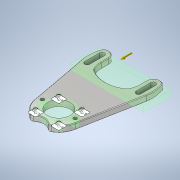
# Autodesk Inventor part: Motor Holder v3
Saved by Autodesk Inventor 2020.1 (Build 241239000, 239)
## iProperties
Created: 2019-03-01
Part Number: Motor Holder v3
Material: Aluminum 6061-AHC
Document SubType Name: Modeling
Designer: Petar
Density: 2.7 g/cm^3
Appearance: Aluminum - Dark
Mass: 29.5264 g
Surface Area: 65.3151 cm^2
Volume: 10.9357 cm^3
Author: Petar
Autodesk Inventor part; units mm, degrees
ref_plane "YZ Plane" through (0, 0, 0) normal (1, 0, 0) x (0, 1, 0)
ref_plane "XZ Plane" through (0, 0, 0) normal (0, 1, 0) x (-1, 0, 0)
ref_plane "XY Plane" through (0, 0, 0) normal (0, 0, 1) x (1, 0, 0)
sketch "Sketch1" plane through (0, 0, 0) normal (0, 1, 0) x (-1, 0, 0)
  line L0 (0, 0) -> (0, 51.5) construction
  circle A0 centre (0, 51.5) radius 9.5
  line L1 (16, -6.25) -> (16, 0)
  line L2 (21.5, 19.9197) -> (21.5, -14.0803) construction
  line L3 (-21.5, 18) -> (-21.5, -16) construction
  circle A1 centre (21.5, 3.5) radius 1.75 construction
  circle A2 centre (21.5, -3.5) radius 1.75 construction
  circle A3 centre (-21.5, 3.5) radius 1.75 construction
  circle A4 centre (-21.5, -3.5) radius 1.75 construction
  line L4 (-16, -6.25) -> (-16, 0)
  line L5 (21.5, 6.25) -> (21.5, -6.25) construction
  line L6 (19.45, 6.25) -> (19.45, -6.25)
  line L7 (23.55, -6.25) -> (23.55, 6.25)
  arc A5 (23.55, 6.25) -> (19.45, 6.25) centre (21.5, 6.25) ccw
  arc A6 (19.45, -6.25) -> (23.55, -6.25) centre (21.5, -6.25) ccw
  line L8 (-19.45, 6.25) -> (-19.45, -6.25)
  line L9 (-23.55, -6.25) -> (-23.55, 6.25)
  arc A7 (-19.45, 6.25) -> (-23.55, 6.25) centre (-21.5, 6.25) ccw
  arc A8 (-23.55, -6.25) -> (-19.45, -6.25) centre (-21.5, -6.25) ccw
  arc A9 (14.5447, 41.7686) -> (17.1997, 54.7282) centre (0, 51.5) ccw construction
  arc A10 (16, -6.25) -> (24.816, -10.638) centre (21.5, -6.25) ccw
  arc A11 (-24.816, -10.638) -> (-16, -6.25) centre (-21.5, -6.25) ccw
  line L10 (17.1997, 54.7282) -> (26.5367, 4.9806)
  line L11 (-17.1997, 54.7282) -> (-26.5367, 4.9806)
  circle A12 centre (0, 51.5) radius 13.75 construction
  circle A13 centre (9.7227, 61.2227) radius 1.5
  circle A14 centre (9.7227, 41.7773) radius 1.5
  line L12 (0, 51.5) -> (9.7227, 61.2227) construction
  line L13 (9.7227, 41.7773) -> (0, 51.5) construction
  circle A15 centre (-9.7227, 61.2227) radius 1.5
  circle A16 centre (-9.7227, 41.7773) radius 1.5
  circle A17 centre (13.75, 51.5) radius 1.5
  line L14 (13.75, 51.5) -> (0, 51.5) construction
  circle A18 centre (-13.75, 51.5) radius 1.5
  circle A19 centre (0, 22.9421) radius 1.5 construction
  line L15 (14.5447, 41.7686) -> (18.7351, 19.4421) construction
  arc A20 (17.1997, 54.7282) -> (-17.1997, 54.7282) centre (0, 51.5) ccw
  arc A21 (-17.1997, 54.7282) -> (-14.5447, 41.7686) centre (0, 51.5) ccw construction
  line L16 (-14.5447, 41.7686) -> (-18.7351, 19.4421) construction
  line L17 (7.5, 67.3114) -> (0, 61) construction
  line L18 (0, 61) -> (-7.5, 67.3114) construction
  spline S0 degree 2 poles (7.5, 67.3114) (0, 61) (-7.5, 67.3114) knots 1 1 1 2 2 2
  line L19 (7.5, 67.3114) -> (-7.5, 67.3114) construction
  line L20 (18.7351, 19.4421) -> (-18.7351, 19.4421) construction
  line L21 (18.7351, 19.4421) -> (11.8062, 33.8844) construction
  line L22 (14.5447, 41.7686) -> (12.1087, 38.1277) construction
  arc A22 (12.1087, 38.1277) -> (11.8062, 33.8844) centre (15.676, 35.7409) ccw construction
  line L23 (-18.7351, 19.4421) -> (-11.8062, 33.8844) construction
  line L24 (-14.5447, 41.7686) -> (-12.1087, 38.1277) construction
  arc A23 (-11.8062, 33.8844) -> (-12.1087, 38.1277) centre (-15.676, 35.7409) ccw construction
  line L25 (14.2986, 19.4421) -> (8.1631, 32.2306) construction
  line L26 (14.2986, 19.4421) -> (7.4946, 25.939) construction
  line L27 (8.1631, 32.2306) -> (6.9952, 30.485) construction
  arc A24 (6.9952, 30.485) -> (7.4946, 25.939) centre (9.9486, 28.509) ccw construction
  line L28 (-14.2986, 19.4421) -> (-8.1631, 32.2306) construction
  line L29 (-14.2986, 19.4421) -> (-7.4946, 25.939) construction
  line L30 (-8.1631, 32.2306) -> (-6.9952, 30.485) construction
  arc A25 (-7.4946, 25.939) -> (-6.9952, 30.485) centre (-9.9486, 28.509) ccw construction
  arc A26 (24.816, -10.638) -> (27, 0) centre (0, 0) ccw
  arc A27 (-24.816, -10.638) -> (24.816, -10.638) centre (0, 0) ccw construction
  arc A28 (-10.2709, 24.9702) -> (-26.5367, 4.9806) centre (0, 0) ccw construction
  line L31 (21.5, -11.75) -> (-21.5, -11.75) construction
  line L32 (-21.2132, 69) -> (25, 69) construction
  line L33 (0, 61) -> (0, 61) construction
  arc A29 (13.761, 8.163) -> (-13.761, 8.163) centre (0, -11.5) ccw
  line L34 (13.761, 8.163) -> (-13.761, 8.163) construction
  arc A30 (16, 0) -> (13.761, 8.163) centre (0, 0) ccw
  arc A31 (-13.761, 8.163) -> (-16, 0) centre (0, 0) ccw
  arc A32 (27, 0) -> (26.5367, 4.9806) centre (0, 0) ccw
  arc A33 (-27, 0) -> (-24.816, -10.638) centre (0, 0) ccw
  arc A34 (-26.5367, 4.9806) -> (-27, 0) centre (0, 0) ccw
  arc A35 (26.5367, 4.9806) -> (-12.0292, 24.1722) centre (0, 0) ccw construction
  line L35 (16, 0) -> (-16, 0) construction
  point P0 (21.5, 0)
  point P1 (0, 12.5)
  dimension "d1" = 19
  dimension "d0" = 51.5
  dimension "d3" = 3.5
  dimension "d4" = 3.5
  dimension "d5" = 7
  dimension "d9" = 3.5
  dimension "d11" = 32
  dimension "d15" = 4.1
  dimension "d24" = 3
  dimension "d25" = 3
  dimension "d27" = 45
  dimension "d29" = 3
  dimension "d30" = 3
  dimension "d50" = 15
  dimension "d53" = 27
  dimension "d75" = 80.75
  dimension "d76" = 8
  dimension "d78" = 0
  dimension "d81" = 6.25
  dimension "d82" = 12.5
  dimension "d85" = 5
  dimension "d86" = 4
  dimension "d98" = 15
  dimension "d99" = 24
  dimension "d101" = 43
  dimension "d104" = 2
  dimension "d105" = 27.5
  constraints: 70 end point, 58 point on circle, 35 centre point, 26 symmetric about line, 19 tangent, 13 point on line, 7 coincident, 5 horizontal, 5 vertical, 3 parallel, 2 perpendicular, 1 collinear, 1 midpoint, 1 vertical alignment, 16 other
  measures "d0" distance of L0.start L0.end
  measures "d3" diameter of A1
  measures "d4" diameter of A2
  measures "d5" distance of A2.centre A1.centre
  measures "d9" vertical distance of L0.start A1.centre
  measures "d11" distance between parallel lines of L4 L1
  measures "d15" distance between parallel lines of L6 L7
  measures "d24" diameter of A13
  measures "d25" diameter of A14
  measures "d27" angle of L0 L13
  measures "d29" diameter of A17
  measures "d30" diameter of A19
  measures "d50" distance of L17.start L18.end
  measures "d53" radius of A26
  measures "d75" distance between parallel lines of L31 L32
  measures "d78" distance of L33.start L33.end
  measures "d81" vertical distance of L5.start point (0, 12.5)
  measures "d82" distance of L5.end L5.start
  measures "d85" distance between parallel lines of L10 L15
  measures "d86" distance between parallel lines of L21 L25
  measures "d98" angle of L15 L21
  measures "d99" radius of A29
  measures "d101" distance of A4.centre A2.centre
  measures "d104" distance edge to line of A19 L20
  measures "d105" diameter of A12
extrude "Extrusion3" add sketch "Sketch1" along normal blind 5 contours L1 A30 A29 A31 L4 A11 A33 A34 L11 A20 S0 L10 A32 A26 A10
thread "Thread1" size "M3x0.5" class "6H" standard "ANSI Metric M Profile" full length
thread "Thread2" size "M3x0.5" class "6H" standard "ANSI Metric M Profile" full length
thread "Thread4" size "M3x0.5" class "6H" standard "ANSI Metric M Profile" full length
thread "Thread5" size "M3x0.5" class "6H" standard "ANSI Metric M Profile" full length
thread "Thread6" size "M3x0.5" class "6H" standard "ANSI Metric M Profile" full length
thread "Thread7" size "M3x0.5" class "6H" standard "ANSI Metric M Profile" full length
sketch "Sketch3" plane through (0, 5, 0) normal (0, 1, 0) x (1, 0, 0)
  line L0 (0, 0) -> (0, -51.5) construction
  circle A0 centre (0, -51.5) radius 9.5 construction
  arc A1 (-24.816, 10.638) -> (-26.5367, -4.9806) centre (0, 0) ccw construction
  line L1 (-7.003, -18.2122) -> (-6.6985, -18.2122)
  line L2 (-7.003, -14.735) -> (-7.003, -18.2122)
  line L3 (-6.6985, -18.2122) -> (-6.6985, -14.735)
  spline S0 degree 3 poles (-5.654, -15.6487) (-5.6375, -15.9355) (-5.5157, -16.1411) (-5.2606, -16.3086) knots 0 0 0 0 1 1 1 1
  spline S1 degree 3 poles (-5.0436, -16.0662) (-5.3012, -15.8898) (-5.3888, -15.6005) (-5.2759, -15.2997) knots 0 0 0 0 1 1 1 1
  spline S2 degree 3 poles (-5.2759, -15.2997) (-5.2175, -15.1423) (-5.0411, -15.0078) (-4.8266, -14.9558) knots 0 0 0 0 1 1 1 1
  spline S3 degree 3 poles (-4.8583, -14.6842) (-5.3723, -14.768) (-5.6832, -15.1436) (-5.654, -15.6487) knots 0 0 0 0 1 1 1 1
  spline S4 degree 3 poles (-4.7441, -14.6652) (-4.7543, -14.6677) (-4.8063, -14.6766) (-4.8583, -14.6842) knots 0 0 0 0 1 1 1 1
  line L4 (-6.6985, -14.735) -> (-7.003, -14.735)
  line L5 (-9.7696, -16.702) -> (-9.4485, -16.702)
  spline S5 degree 3 poles (-9.4485, -16.702) (-8.9497, -16.702) (-8.6731, -16.669) (-8.4294, -16.5814) knots 0 0 0 0 1 1 1 1
  line L6 (-10.0741, -14.7324) -> (-10.0741, -18.2122)
  line L7 (-9.7696, -18.2122) -> (-9.7696, -16.702)
  line L8 (-10.0741, -18.2122) -> (-9.7696, -18.2122)
  spline S6 degree 3 poles (-7.8457, -15.9418) (-7.8165, -15.7946) (-7.8266, -15.5193) (-7.866, -15.3822) knots 0 0 0 0 1 1 1 1
  spline S7 degree 3 poles (-8.4294, -16.5814) (-8.1084, -16.4672) (-7.9066, -16.2464) (-7.8457, -15.9418) knots 0 0 0 0 1 1 1 1
  spline S8 degree 3 poles (-7.866, -15.3822) (-7.965, -15.0383) (-8.1997, -14.8543) (-8.6439, -14.7718) knots 0 0 0 0 1 1 1 1
  spline S9 degree 3 poles (-8.1617, -15.6487) (-8.1426, -15.9609) (-8.2568, -16.1868) (-8.4916, -16.301) knots 0 0 0 0 1 1 1 1
  spline S10 degree 3 poles (-8.6236, -15.0624) (-8.3178, -15.1462) (-8.1832, -15.3187) (-8.1617, -15.6487) knots 0 0 0 0 1 1 1 1
  spline S11 degree 3 poles (-8.4916, -16.301) (-8.6782, -16.3936) (-8.8127, -16.4101) (-9.366, -16.4101) knots 0 0 0 0 1 1 1 1
  line L9 (-9.366, -16.4101) -> (-9.7696, -16.4101)
  line L10 (-9.7696, -16.4101) -> (-9.7696, -15.0243)
  spline S12 degree 3 poles (-4.5284, -16.301) (-4.6305, -16.2646) (-4.7394, -16.2225) (-4.9041, -16.1474) (-4.9836, -16.1078) (-5.0436, -16.0662) knots -1.508252 -1.508252 -1.508252 -1.508252 -0.608749 -0.608749 0 0 0 0
  spline S13 degree 3 poles (-5.2606, -16.3086) (-5.1261, -16.3974) (-4.9599, -16.4698) (-4.5982, -16.5954) knots 0 0 0 0 1 1 1 1
  line L11 (-5.4078, -17.3111) -> (-5.7353, -17.3111)
  line L12 (-5.7353, -17.3111) -> (-5.7264, -17.3708)
  line L13 (-5.3875, -17.4101) -> (-5.4078, -17.3111)
  spline S14 degree 3 poles (-4.8266, -14.9558) (-4.7061, -14.9253) (-4.4205, -14.9266) (-4.2809, -14.9558) knots 0 0 0 0 1 1 1 1
  spline S15 degree 3 poles (-4.2289, -14.6893) (-4.3215, -14.6715) (-4.6972, -14.6538) (-4.7441, -14.6652) knots 0 0 0 0 1 1 1 1
  line L14 (-3.8012, -15.405) -> (-3.786, -15.4837)
  spline S16 degree 3 poles (-4.2809, -14.9558) (-4.0106, -15.0142) (-3.8469, -15.169) (-3.8012, -15.405) knots 0 0 0 0 1 1 1 1
  line L15 (-3.786, -15.4837) -> (-3.4738, -15.4837)
  line L16 (-3.4738, -15.4837) -> (-3.4827, -15.4355)
  spline S17 degree 3 poles (-3.4827, -15.4355) (-3.5233, -15.1982) (-3.5817, -15.07) (-3.7086, -14.9431) knots 0 0 0 0 1 1 1 1
  spline S18 degree 3 poles (-3.7086, -14.9431) (-3.8456, -14.8073) (-3.9903, -14.7363) (-4.2289, -14.6893) knots 0 0 0 0 1 1 1 1
  spline S19 degree 3 poles (-1.4344, -14.6779) (-1.8812, -14.7502) (-2.2187, -15.0066) (-2.4281, -15.4304) knots 0 0 0 0 1 1 1 1
  spline S20 degree 3 poles (-2.3202, -16.4736) (-2.3202, -15.683) (-2.0144, -15.1373) (-1.4877, -14.9863) knots 0 0 0 0 1 1 1 1
  spline S21 degree 3 poles (-1.4877, -14.9863) (-1.4027, -14.9621) (-1.357, -14.9571) (-1.1908, -14.9571) knots 0 0 0 0 1 1 1 1
  spline S22 degree 3 poles (-1.1908, -14.9571) (-1.0195, -14.9571) (-0.9814, -14.9609) (-0.8989, -14.9863) knots 0 0 0 0 1 1 1 1
  spline S23 degree 3 poles (-0.8532, -14.6956) (-0.9916, -14.6614) (-1.2834, -14.6525) (-1.4344, -14.6779) knots 0 0 0 0 1 1 1 1
  line L17 (-0.3862, -15.5116) -> (-0.3786, -15.5472)
  spline S24 degree 3 poles (-0.8989, -14.9863) (-0.6121, -15.0776) (-0.4446, -15.2489) (-0.3862, -15.5116) knots 0 0 0 0 1 1 1 1
  spline S25 degree 3 poles (-0.1882, -15.1233) (-0.3266, -14.9127) (-0.5461, -14.7705) (-0.8532, -14.6956) knots 0 0 0 0 1 1 1 1
  spline S26 degree 3 poles (-0.0537, -15.4812) (-0.069, -15.3708) (-0.1261, -15.2185) (-0.1882, -15.1233) knots 0 0 0 0 1 1 1 1
  line L18 (-0.3786, -15.5472) -> (-0.0448, -15.5472)
  line L19 (-0.0448, -15.5472) -> (-0.0537, -15.4812)
  spline S27 degree 3 poles (-2.4281, -15.4304) (-2.6451, -15.8695) (-2.7086, -16.4774) (-2.5944, -17.0332) knots 0 0 0 0 1 1 1 1
  spline S28 degree 3 poles (-5.2365, -17.7401) (-5.3, -17.6614) (-5.3634, -17.5231) (-5.3875, -17.4101) knots 0 0 0 0 1 1 1 1
  spline S29 degree 3 poles (-5.7264, -17.3708) (-5.6997, -17.5535) (-5.6071, -17.7794) (-5.5056, -17.9051) knots 0 0 0 0 1 1 1 1
  spline S30 degree 3 poles (-4.7746, -17.9914) (-4.8679, -17.9737) (-4.9599, -17.9443) (-5.1175, -17.8586) (-5.1837, -17.8061) (-5.2365, -17.7401) knots -1.494677 -1.494677 -1.494677 -1.494677 -0.705114 -0.705114 0 0 0 0
  spline S31 degree 3 poles (-5.5056, -17.9051) (-5.305, -18.1538) (-4.9561, -18.2883) (-4.5094, -18.2883) knots 0 0 0 0 1 1 1 1
  spline S32 degree 3 poles (-9.2454, -15.0294) (-8.7581, -15.0345) (-8.7162, -15.037) (-8.6236, -15.0624) knots 0 0 0 0 1 1 1 1
  spline S33 degree 3 poles (-8.6439, -14.7718) (-8.7721, -14.7477) (-8.847, -14.7439) (-9.4294, -14.7388) knots 0 0 0 0 1 1 1 1
  line L20 (-9.4294, -14.7388) -> (-10.0741, -14.7324)
  line L21 (-9.7696, -15.0243) -> (-9.2454, -15.0294)
  spline S34 degree 3 poles (-0.7314, -17.8936) (-0.8862, -17.9711) (-0.9751, -17.9901) (-1.1908, -17.9901) knots 0 0 0 0 1 1 1 1
  spline S35 degree 3 poles (-0.3862, -17.4342) (-0.4306, -17.6373) (-0.5588, -17.8061) (-0.7314, -17.8936) knots 0 0 0 0 1 1 1 1
  spline S36 degree 3 poles (-1.1083, -18.2832) (-0.6997, -18.2629) (-0.3672, -18.0967) (-0.1882, -17.8238) knots 0 0 0 0 1 1 1 1
  line L22 (-0.3786, -17.4) -> (-0.3862, -17.4342)
  line L23 (-0.0461, -17.4) -> (-0.3786, -17.4)
  line L24 (-0.055, -17.466) -> (-0.0461, -17.4)
  spline S37 degree 3 poles (-0.1882, -17.8238) (-0.1261, -17.7287) (-0.0702, -17.5776) (-0.055, -17.466) knots 0 0 0 0 1 1 1 1
  line L25 (1.1569, -14.735) -> (0.8524, -14.735)
  line L26 (1.1569, -16.2578) -> (1.1569, -14.735)
  line L27 (0.8524, -14.735) -> (0.8524, -18.2122)
  line L28 (0.8524, -18.2122) -> (1.1569, -18.2122)
  line L29 (1.1569, -18.2122) -> (1.1569, -16.5497)
  line L30 (1.1569, -16.5497) -> (3.0224, -16.5497)
  line L31 (3.0224, -16.2578) -> (1.1569, -16.2578)
  line L32 (5.1786, -16.4025) -> (5.9413, -15.5751)
  line L33 (4.8055, -16.3543) -> (4.8017, -15.5446)
  spline S38 degree 3 poles (6.7027, -14.7413) (6.7027, -14.7375) (6.6177, -14.735) (6.5149, -14.735) knots 0 0 0 0 1 1 1 1
  spline S39 degree 3 poles (5.9413, -15.5751) (6.36, -15.1195) (6.7027, -14.7439) (6.7027, -14.7413) knots 0 0 0 0 1 1 1 1
  line L34 (6.5149, -14.735) -> (6.3258, -14.735)
  line L35 (6.3258, -14.735) -> (4.8055, -16.3543)
  line L36 (4.8017, -15.5446) -> (4.7991, -14.735)
  line L37 (3.327, -14.735) -> (3.0224, -14.735)
  line L38 (4.7991, -14.735) -> (4.4945, -14.735)
  line L39 (3.0224, -14.735) -> (3.0224, -16.2578)
  line L40 (5.2344, -16.4596) -> (5.1786, -16.4025)
  spline S40 degree 3 poles (6.0174, -17.3048) (5.6176, -16.8721) (5.2649, -16.4913) (5.2344, -16.4596) knots 0 0 0 0 1 1 1 1
  line L41 (4.8017, -17.3568) -> (4.8055, -16.5002)
  line L42 (4.4945, -14.735) -> (4.4945, -18.2122)
  line L43 (3.327, -18.2122) -> (3.327, -14.735)
  line L44 (4.8055, -16.5002) -> (6.4298, -18.2109)
  line L45 (3.0224, -16.5497) -> (3.0224, -18.2122)
  line L46 (3.0224, -18.2122) -> (3.327, -18.2122)
  line L47 (4.4945, -18.2122) -> (4.7991, -18.2122)
  line L48 (4.7991, -18.2122) -> (4.8017, -17.3568)
  line L49 (6.4298, -18.2109) -> (6.6456, -18.2122)
  spline S41 degree 3 poles (6.8029, -18.1513) (6.7699, -18.1183) (6.4171, -17.7375) (6.0174, -17.3048) knots 0 0 0 0 1 1 1 1
  line L50 (6.86, -18.2122) -> (6.8029, -18.1513)
  line L51 (6.6456, -18.2122) -> (6.86, -18.2122)
  spline S42 degree 3 poles (8.3892, -14.7629) (8.3829, -14.7794) (8.0783, -15.5599) (7.7116, -16.499) knots 0 0 0 0 1 1 1 1
  spline S43 degree 3 poles (8.1976, -16.0053) (8.5695, -15.0345) (8.5745, -15.0243) (8.591, -15.0662) knots 0 0 0 0 1 1 1 1
  spline S44 degree 3 poles (8.5796, -14.735) (8.4083, -14.735) (8.4019, -14.7363) (8.3892, -14.7629) knots 0 0 0 0 1 1 1 1
  line L52 (8.756, -14.735) -> (8.5796, -14.735)
  line L53 (8.8524, -14.9786) -> (8.756, -14.735)
  spline S45 degree 3 poles (8.591, -15.0662) (8.6012, -15.089) (8.8182, -15.6652) (9.0758, -16.3467) knots 0 0 0 0 1 1 1 1
  spline S46 degree 3 poles (9.5314, -16.7147) (9.2103, -15.8949) (8.9057, -15.1132) (8.8524, -14.9786) knots 0 0 0 0 1 1 1 1
  spline S47 degree 3 poles (7.7573, -17.1652) (7.7915, -17.0675) (7.9908, -16.5459) (8.1976, -16.0053) knots 0 0 0 0 1 1 1 1
  line L54 (7.0479, -18.2058) -> (7.2001, -18.2096)
  spline S48 degree 3 poles (7.2001, -18.2096) (7.2839, -18.2109) (7.3562, -18.2109) (7.3588, -18.2071) knots 0 0 0 0 1 1 1 1
  line L55 (7.7116, -16.499) -> (7.0479, -18.2058)
  spline S49 degree 3 poles (7.3588, -18.2071) (7.3677, -18.1982) (7.6824, -17.3746) (7.7573, -17.1652) knots 0 0 0 0 1 1 1 1
  spline S50 degree 3 poles (-4.1934, -17.9774) (-4.3101, -18.0104) (-4.6324, -18.018) (-4.7746, -17.9914) knots 0 0 0 0 1 1 1 1
  ellipse E0 centre (-21.8716, 1.388) end of major axis (-3.6125, -17.9928) minor radius 4.9544 (-4.5094, -18.2883) -> (-3.8558, -18.1589) ccw
  spline S51 degree 3 poles (-3.8558, -18.1589) (-3.7695, -18.117) (-3.7276, -18.0865) (-3.6451, -18.004) knots 0 0 0 0 1 1 1 1
  spline S52 degree 3 poles (-3.7327, -17.3924) (-3.753, -17.7084) (-3.9015, -17.8962) (-4.1934, -17.9774) knots 0 0 0 0 1 1 1 1
  spline S53 degree 3 poles (-3.6451, -18.004) (-3.4789, -17.8378) (-3.4154, -17.6779) (-3.4027, -17.3924) knots 0 0 0 0 1 1 1 1
  spline S54 degree 3 poles (-4.5982, -16.5954) (-4.2644, -16.7109) (-4.1464, -16.7604) (-4.0284, -16.834) knots 0 0 0 0 1 1 1 1
  spline S55 degree 3 poles (-3.951, -16.5281) (-4.0626, -16.4723) (-4.1743, -16.4292) (-4.5284, -16.301) knots 0 0 0 0 1 1 1 1
  spline S56 degree 3 poles (-1.1908, -17.9901) (-1.357, -17.9901) (-1.4027, -17.985) (-1.4877, -17.9609) knots 0 0 0 0 1 1 1 1
  spline S57 degree 3 poles (-1.4877, -17.9609) (-2.0144, -17.8099) (-2.3202, -17.2629) (-2.3202, -16.4736) knots 0 0 0 0 1 1 1 1
  spline S58 degree 3 poles (-2.5944, -17.0332) (-2.423, -17.8632) (-1.8761, -18.3226) (-1.1083, -18.2832) knots 0 0 0 0 1 1 1 1
  spline S59 degree 3 poles (-3.4167, -17.1297) (-3.4751, -16.8683) (-3.6413, -16.6817) (-3.951, -16.5281) knots 0 0 0 0 1 1 1 1
  spline S60 degree 3 poles (-4.0284, -16.834) (-3.8076, -16.971) (-3.7162, -17.1449) (-3.7327, -17.3924) knots 0 0 0 0 1 1 1 1
  spline S61 degree 3 poles (-3.4027, -17.3924) (-3.3977, -17.2617) (-3.4002, -17.2058) (-3.4167, -17.1297) knots 0 0 0 0 1 1 1 1
  line L56 (8.204, -17.9203) -> (8.1532, -18.0637)
  line L57 (8.1532, -18.0637) -> (8.1037, -18.2058)
  line L58 (8.1037, -18.2058) -> (8.6012, -18.2096)
  line L59 (8.9362, -17.9178) -> (8.204, -17.9203)
  spline S62 degree 3 poles (9.0758, -16.3467) (9.3334, -17.0269) (9.572, -17.6576) (9.6063, -17.749) knots 0 0 0 0 1 1 1 1
  line L60 (9.6697, -17.9139) -> (8.9362, -17.9178)
  spline S63 degree 3 poles (8.6012, -18.2096) (8.8753, -18.2109) (9.3271, -18.2109) (9.6063, -18.2096) knots 0 0 0 0 1 1 1 1
  line L61 (9.6063, -17.749) -> (9.6697, -17.9139)
  line L62 (9.6063, -18.2096) -> (10.1139, -18.2058)
  line L63 (10.1139, -18.2058) -> (9.5314, -16.7147)
  point P0 (0, -22.9421)
  constraints: 128 end point, 2 coincident, 2 horizontal alignment, 1 vertical, 194 other
emboss "Emboss1" [suppressed]
sketch "Sketch4" plane through (0, 0, 0) normal (0, -1, 0) x (1, 0, 0)
  circle A0 centre (0, 51.5) radius 9.5 construction
  arc A1 (24.816, -10.638) -> (26.5367, 4.9806) centre (0, 0) ccw construction
  line L0 (0, 0) -> (0, 51.5) construction
  spline S0 degree 3 poles (8.013, 15.7172) (7.9838, 15.57) (7.994, 15.2946) (8.0333, 15.1575) knots 0 0 0 0 1 1 1 1
  spline S1 degree 3 poles (8.5968, 16.3568) (8.2757, 16.2425) (8.0739, 16.0217) (8.013, 15.7172) knots 0 0 0 0 1 1 1 1
  spline S2 degree 3 poles (8.329, 15.424) (8.31, 15.7362) (8.4242, 15.9621) (8.6589, 16.0763) knots 0 0 0 0 1 1 1 1
  spline S3 degree 3 poles (8.7909, 14.8377) (8.4851, 14.9215) (8.3506, 15.0941) (8.329, 15.424) knots 0 0 0 0 1 1 1 1
  spline S4 degree 3 poles (8.0333, 15.1575) (8.1323, 14.8136) (8.3671, 14.6296) (8.8112, 14.5471) knots 0 0 0 0 1 1 1 1
  spline S5 degree 3 poles (9.6158, 16.4773) (9.1171, 16.4773) (8.8404, 16.4443) (8.5968, 16.3568) knots 0 0 0 0 1 1 1 1
  line L1 (9.9369, 16.4773) -> (9.6158, 16.4773)
  line L2 (9.9369, 17.9875) -> (9.9369, 16.4773)
  line L3 (10.2414, 17.9875) -> (9.9369, 17.9875)
  line L4 (10.2414, 14.5078) -> (10.2414, 17.9875)
  spline S6 degree 3 poles (8.6589, 16.0763) (8.8455, 16.1689) (8.98, 16.1854) (9.5333, 16.1854) knots 0 0 0 0 1 1 1 1
  line L5 (9.5333, 16.1854) -> (9.9369, 16.1854)
  spline S7 degree 3 poles (9.4128, 14.8047) (8.9254, 14.8098) (8.8836, 14.8123) (8.7909, 14.8377) knots 0 0 0 0 1 1 1 1
  line L6 (9.9369, 16.1854) -> (9.9369, 14.7996)
  spline S8 degree 3 poles (8.8112, 14.5471) (8.9394, 14.523) (9.0143, 14.5192) (9.5968, 14.5141) knots 0 0 0 0 1 1 1 1
  line L7 (9.9369, 14.7996) -> (9.4128, 14.8047)
  line L8 (9.5968, 14.5141) -> (10.2414, 14.5078)
  spline S9 degree 3 poles (4.9114, 14.4405) (4.9216, 14.443) (4.9736, 14.4519) (5.0257, 14.4595) knots 0 0 0 0 1 1 1 1
  spline S10 degree 3 poles (4.9939, 14.7311) (4.8734, 14.7007) (4.5878, 14.7019) (4.4482, 14.7311) knots 0 0 0 0 1 1 1 1
  spline S11 degree 3 poles (3.8759, 14.7184) (4.013, 14.5826) (4.1576, 14.5116) (4.3962, 14.4646) knots 0 0 0 0 1 1 1 1
  spline S12 degree 3 poles (4.3962, 14.4646) (4.4889, 14.4468) (4.8645, 14.4291) (4.9114, 14.4405) knots 0 0 0 0 1 1 1 1
  spline S13 degree 3 poles (4.4482, 14.7311) (4.1779, 14.7895) (4.0142, 14.9443) (3.9685, 15.1804) knots 0 0 0 0 1 1 1 1
  line L9 (3.9685, 15.1804) -> (3.9533, 15.259)
  spline S14 degree 3 poles (4.1183, 16.3035) (4.23, 16.2476) (4.3416, 16.2045) (4.6957, 16.0763) knots 0 0 0 0 1 1 1 1
  spline S15 degree 3 poles (4.7655, 16.3707) (4.4317, 16.4862) (4.3137, 16.5357) (4.1957, 16.6093) knots 0 0 0 0 1 1 1 1
  line L10 (3.9533, 15.259) -> (3.6411, 15.259)
  line L11 (3.6411, 15.259) -> (3.65, 15.2108)
  spline S16 degree 3 poles (3.584, 16.905) (3.6424, 16.6436) (3.8086, 16.457) (4.1183, 16.3035) knots 0 0 0 0 1 1 1 1
  spline S17 degree 3 poles (4.1957, 16.6093) (3.9749, 16.7464) (3.8835, 16.9202) (3.9, 17.1677) knots 0 0 0 0 1 1 1 1
  spline S18 degree 3 poles (3.5701, 17.1677) (3.565, 17.037) (3.5675, 16.9811) (3.584, 16.905) knots 0 0 0 0 1 1 1 1
  spline S19 degree 3 poles (1.6018, 14.4532) (2.0485, 14.5255) (2.386, 14.7819) (2.5954, 15.2057) knots 0 0 0 0 1 1 1 1
  spline S20 degree 3 poles (2.5954, 15.2057) (2.8124, 15.6448) (2.8759, 16.2527) (2.7617, 16.8085) knots 0 0 0 0 1 1 1 1
  spline S21 degree 3 poles (2.4876, 16.2489) (2.4876, 15.4583) (2.1817, 14.9126) (1.6551, 14.7616) knots 0 0 0 0 1 1 1 1
  spline S22 degree 3 poles (3.8125, 17.7794) (3.6462, 17.6131) (3.5828, 17.4532) (3.5701, 17.1677) knots 0 0 0 0 1 1 1 1
  spline S23 degree 3 poles (1.6551, 17.7362) (2.1817, 17.5852) (2.4876, 17.0382) (2.4876, 16.2489) knots 0 0 0 0 1 1 1 1
  spline S24 degree 3 poles (1.3581, 17.7654) (1.5244, 17.7654) (1.57, 17.7603) (1.6551, 17.7362) knots 0 0 0 0 1 1 1 1
  spline S25 degree 3 poles (2.7617, 16.8085) (2.5904, 17.6385) (2.0434, 18.0979) (1.2756, 18.0586) knots 0 0 0 0 1 1 1 1
  spline S26 degree 3 poles (3.65, 15.2108) (3.6906, 14.9735) (3.749, 14.8453) (3.8759, 14.7184) knots 0 0 0 0 1 1 1 1
  line L12 (0.5459, 15.3225) -> (0.2122, 15.3225)
  line L13 (0.5535, 15.287) -> (0.5459, 15.3225)
  line L14 (0.2122, 15.3225) -> (0.221, 15.2565)
  spline S27 degree 3 poles (0.221, 15.2565) (0.2363, 15.1461) (0.2934, 14.9938) (0.3556, 14.8986) knots 0 0 0 0 1 1 1 1
  spline S28 degree 3 poles (1.0662, 14.7616) (0.7794, 14.8529) (0.6119, 15.0243) (0.5535, 15.287) knots 0 0 0 0 1 1 1 1
  spline S29 degree 3 poles (0.3556, 14.8986) (0.4939, 14.688) (0.7134, 14.5458) (1.0205, 14.471) knots 0 0 0 0 1 1 1 1
  line L15 (-0.9896, 16.0332) -> (-0.9896, 14.5103)
  line L16 (-0.9896, 14.5103) -> (-0.6851, 14.5103)
  spline S30 degree 3 poles (1.6551, 14.7616) (1.57, 14.7375) (1.5244, 14.7324) (1.3581, 14.7324) knots 0 0 0 0 1 1 1 1
  spline S31 degree 3 poles (1.3581, 14.7324) (1.1868, 14.7324) (1.1487, 14.7362) (1.0662, 14.7616) knots 0 0 0 0 1 1 1 1
  spline S32 degree 3 poles (1.0205, 14.471) (1.1589, 14.4367) (1.4508, 14.4278) (1.6018, 14.4532) knots 0 0 0 0 1 1 1 1
  line L17 (-0.6851, 14.5103) -> (-0.6851, 17.9875)
  line L18 (0.2134, 17.1753) -> (0.5459, 17.1753)
  line L19 (0.5459, 17.1753) -> (0.5535, 17.2096)
  line L20 (0.2223, 17.2413) -> (0.2134, 17.1753)
  line L21 (-0.9896, 17.9875) -> (-0.9896, 16.325)
  line L22 (-0.6851, 17.9875) -> (-0.9896, 17.9875)
  spline S33 degree 3 poles (0.5535, 17.2096) (0.598, 17.4126) (0.7261, 17.5814) (0.8987, 17.669) knots 0 0 0 0 1 1 1 1
  spline S34 degree 3 poles (0.8987, 17.669) (1.0535, 17.7464) (1.1424, 17.7654) (1.3581, 17.7654) knots 0 0 0 0 1 1 1 1
  spline S35 degree 3 poles (1.2756, 18.0586) (0.867, 18.0383) (0.5345, 17.872) (0.3556, 17.5992) knots 0 0 0 0 1 1 1 1
  spline S36 degree 3 poles (0.3556, 17.5992) (0.2934, 17.504) (0.2375, 17.353) (0.2223, 17.2413) knots 0 0 0 0 1 1 1 1
  line L23 (7.1704, 17.9875) -> (6.8658, 17.9875)
  line L24 (7.1704, 14.5103) -> (7.1704, 17.9875)
  line L25 (6.8658, 17.9875) -> (6.8658, 14.5103)
  spline S37 degree 3 poles (5.8214, 15.424) (5.8049, 15.7108) (5.683, 15.9164) (5.4279, 16.0839) knots 0 0 0 0 1 1 1 1
  spline S38 degree 3 poles (5.2109, 15.8415) (5.4686, 15.6651) (5.5561, 15.3758) (5.4432, 15.075) knots 0 0 0 0 1 1 1 1
  line L26 (6.8658, 14.5103) -> (7.1704, 14.5103)
  line L27 (5.9026, 17.0865) -> (5.8937, 17.1461)
  spline S39 degree 3 poles (5.8937, 17.1461) (5.867, 17.3289) (5.7744, 17.5547) (5.6729, 17.6804) knots 0 0 0 0 1 1 1 1
  line L28 (5.5752, 17.0865) -> (5.9026, 17.0865)
  spline S40 degree 3 poles (5.0257, 14.4595) (5.5396, 14.5433) (5.8505, 14.9189) (5.8214, 15.424) knots 0 0 0 0 1 1 1 1
  spline S41 degree 3 poles (5.4432, 15.075) (5.3848, 14.9177) (5.2084, 14.7831) (4.9939, 14.7311) knots 0 0 0 0 1 1 1 1
  line L29 (5.5549, 17.1855) -> (5.5752, 17.0865)
  spline S42 degree 3 poles (5.4038, 17.5154) (5.4673, 17.4367) (5.5307, 17.2984) (5.5549, 17.1855) knots 0 0 0 0 1 1 1 1
  line L30 (-0.9896, 16.325) -> (-2.8551, 16.325)
  line L31 (-2.8551, 16.0332) -> (-0.9896, 16.0332)
  line L32 (-4.6381, 16.1296) -> (-4.6343, 15.32)
  line L33 (-4.6318, 14.5103) -> (-4.3272, 14.5103)
  line L34 (-4.6343, 15.32) -> (-4.6318, 14.5103)
  line L35 (-5.0112, 16.1778) -> (-5.7739, 15.3504)
  line L36 (-6.1585, 14.5103) -> (-4.6381, 16.1296)
  line L37 (-6.3475, 14.5103) -> (-6.1585, 14.5103)
  spline S43 degree 3 poles (-6.5354, 14.5166) (-6.5354, 14.5128) (-6.4503, 14.5103) (-6.3475, 14.5103) knots 0 0 0 0 1 1 1 1
  spline S44 degree 3 poles (-5.7739, 15.3504) (-6.1927, 14.8948) (-6.5354, 14.5192) (-6.5354, 14.5166) knots 0 0 0 0 1 1 1 1
  line L38 (-2.8551, 17.9875) -> (-3.1597, 17.9875)
  line L39 (-2.8551, 16.325) -> (-2.8551, 17.9875)
  line L40 (-2.8551, 14.5103) -> (-2.8551, 16.0332)
  line L41 (-3.1597, 14.5103) -> (-2.8551, 14.5103)
  line L42 (-3.1597, 17.9875) -> (-3.1597, 14.5103)
  line L43 (-4.3272, 14.5103) -> (-4.3272, 17.9875)
  line L44 (-4.3272, 17.9875) -> (-4.6318, 17.9875)
  line L45 (-4.6318, 17.9875) -> (-4.6343, 17.1322)
  line L46 (-4.6343, 17.1322) -> (-4.6381, 16.2755)
  line L47 (-6.8805, 17.9811) -> (-7.0328, 17.985)
  spline S45 degree 3 poles (-7.0328, 17.985) (-7.1166, 17.9862) (-7.1889, 17.9862) (-7.1915, 17.9824) knots 0 0 0 0 1 1 1 1
  spline S46 degree 3 poles (-7.1915, 17.9824) (-7.2003, 17.9735) (-7.5151, 17.1499) (-7.5899, 16.9405) knots 0 0 0 0 1 1 1 1
  spline S47 degree 3 poles (-7.5899, 16.9405) (-7.6242, 16.8428) (-7.8234, 16.3212) (-8.0303, 15.7806) knots 0 0 0 0 1 1 1 1
  line L48 (-7.9859, 17.839) -> (-7.9364, 17.9811)
  line L49 (-8.0366, 17.6956) -> (-7.9859, 17.839)
  line L50 (-7.5443, 16.2743) -> (-6.8805, 17.9811)
  spline S48 degree 3 poles (-8.2219, 14.5382) (-8.2156, 14.5547) (-7.911, 15.3352) (-7.5443, 16.2743) knots 0 0 0 0 1 1 1 1
  spline S49 degree 3 poles (-8.0303, 15.7806) (-8.4021, 14.8098) (-8.4072, 14.7996) (-8.4237, 14.8415) knots 0 0 0 0 1 1 1 1
  spline S50 degree 3 poles (-8.4123, 14.5103) (-8.241, 14.5103) (-8.2346, 14.5116) (-8.2219, 14.5382) knots 0 0 0 0 1 1 1 1
  line L51 (-7.9364, 17.9811) -> (-8.4339, 17.985)
  line L52 (-8.7689, 17.6931) -> (-8.0366, 17.6956)
  line L53 (-8.5887, 14.5103) -> (-8.4123, 14.5103)
  line L54 (-8.6851, 14.754) -> (-8.5887, 14.5103)
  spline S51 degree 3 poles (-8.4237, 14.8415) (-8.4339, 14.8644) (-8.6509, 15.4405) (-8.9085, 16.122) knots 0 0 0 0 1 1 1 1
  spline S52 degree 3 poles (-9.3641, 16.49) (-9.043, 15.6702) (-8.7384, 14.8885) (-8.6851, 14.754) knots 0 0 0 0 1 1 1 1
  spline S53 degree 3 poles (-8.9085, 16.122) (-9.1661, 16.8022) (-9.4047, 17.4329) (-9.4389, 17.5243) knots 0 0 0 0 1 1 1 1
  spline S54 degree 3 poles (-8.4339, 17.985) (-8.708, 17.9862) (-9.1598, 17.9862) (-9.4389, 17.985) knots 0 0 0 0 1 1 1 1
  line L55 (-9.5024, 17.6893) -> (-8.7689, 17.6931)
  line L56 (-9.4389, 17.5243) -> (-9.5024, 17.6893)
  line L57 (-9.9466, 17.9811) -> (-9.3641, 16.49)
  line L58 (-9.4389, 17.985) -> (-9.9466, 17.9811)
  line L59 (-5.0671, 16.2349) -> (-5.0112, 16.1778)
  spline S55 degree 3 poles (-5.8501, 17.0801) (-5.4503, 16.6474) (-5.0975, 16.2667) (-5.0671, 16.2349) knots 0 0 0 0 1 1 1 1
  line L60 (-4.6381, 16.2755) -> (-6.2625, 17.9862)
  spline S56 degree 3 poles (-6.6356, 17.9266) (-6.6026, 17.8936) (-6.2498, 17.5129) (-5.8501, 17.0801) knots 0 0 0 0 1 1 1 1
  line L61 (-6.2625, 17.9862) -> (-6.4783, 17.9875)
  line L62 (-6.6927, 17.9875) -> (-6.6356, 17.9266)
  line L63 (-6.4783, 17.9875) -> (-6.6927, 17.9875)
  spline S57 degree 3 poles (4.6957, 16.0763) (4.7978, 16.0399) (4.9067, 15.9978) (5.0715, 15.9228) (5.1509, 15.8831) (5.2109, 15.8415) knots -1.508252 -1.508252 -1.508252 -1.508252 -0.608749 -0.608749 0 0 0 0
  spline S58 degree 3 poles (5.4279, 16.0839) (5.2934, 16.1728) (5.1272, 16.2451) (4.7655, 16.3707) knots 0 0 0 0 1 1 1 1
  spline S59 degree 3 poles (4.0231, 17.9342) (3.9368, 17.8923) (3.8949, 17.8619) (3.8125, 17.7794) knots 0 0 0 0 1 1 1 1
  spline S60 degree 3 poles (4.3607, 17.7527) (4.4774, 17.7857) (4.7998, 17.7933) (4.9419, 17.7667) knots 0 0 0 0 1 1 1 1
  ellipse E0 centre (22.0389, -1.6127) end of major axis (3.7798, 17.7681) minor radius 4.9544 (4.6767, 18.0636) -> (4.0231, 17.9342) ccw
  spline S61 degree 3 poles (4.9419, 17.7667) (5.0353, 17.7491) (5.1272, 17.7197) (5.2848, 17.6339) (5.351, 17.5814) (5.4038, 17.5154) knots -1.494677 -1.494677 -1.494677 -1.494677 -0.705114 -0.705114 0 0 0 0
  spline S62 degree 3 poles (5.6729, 17.6804) (5.4724, 17.9291) (5.1234, 18.0636) (4.6767, 18.0636) knots 0 0 0 0 1 1 1 1
  spline S63 degree 3 poles (3.9, 17.1677) (3.9203, 17.4837) (4.0688, 17.6715) (4.3607, 17.7527) knots 0 0 0 0 1 1 1 1
  constraints: 128 end point, 2 horizontal alignment, 1 vertical, 194 other
emboss "Emboss2" [suppressed]
fillet "Fillet3" [suppressed]
fillet "Fillet5" radius 2 6 edges at (-7.5, 2.5, 67.3114) (7.5, 2.5, 67.3114) (24.816, 2.5, -10.638) (-24.816, 2.5, -10.638) (-13.761, 2.5, 8.163) (13.761, 2.5, 8.163)
chamfer "Chamfer3" distance 0.5 angle 45 40 edges at (14.2685, 5, 61.6321) (21.8682, 5, 29.8544) (26.5103, 5, -5.1191) (24.7034, 5, -10.6299) (18.713, 5, -10.9916) (16, 5, -3.125) (15.4929, 5, 3.9962) (13.7269, 5, 8.124) (0, 5, 12.5) (7.6088, 5, 66.9375) (0, 5, 64.1557) (-7.6088, 5, 66.9375) (-14.2685, 5, 61.6321) (-21.8682, 5, 29.8544) (-26.8839, 5, 2.501) (-24.7034, 5, -10.6299) (-18.713, 5, -10.9916) (-16, 5, -3.125) (-15.4929, 5, 3.9962) (-13.7269, 5, 8.124) (0, 0, 64.1557) (7.6088, 0, 66.9375) (14.2685, 0, 61.6321) (21.8682, 0, 29.8544) (26.5103, 0, -5.1191) (24.7034, 0, -10.6299) (18.713, 0, -10.9916) (16, 0, -3.125) (15.4929, 0, 3.9962) (13.7269, 0, 8.124) (0, 0, 12.5) (-7.6088, 0, 66.9375) (-14.2685, 0, 61.6321) (-21.8682, 0, 29.8544) (-26.5103, 0, -5.1191) (-24.7034, 0, -10.6299) (-18.713, 0, -10.9916) (-16, 0, -3.125) (-15.4929, 0, 3.9962) (-13.7269, 0, 8.124)
sketch "Center Lines" plane through (0, 5, 0) normal (0, 1, 0) x (1, 0, 0)
  arc A0 (-23.55, -6.25) -> (-19.45, -6.25) centre (-21.5, -6.25) ccw construction
  line L0 (-23.55, -6.25) -> (-23.55, 6.25) construction
  arc A1 (-19.45, 6.25) -> (-23.55, 6.25) centre (-21.5, 6.25) ccw construction
  line L1 (-19.45, 6.25) -> (-19.45, -6.25) construction
  line L2 (-21.5, -6.25) -> (-21.5, 6.25) construction
  line L3 (19.45, -6.25) -> (19.45, 6.25) construction
  arc A2 (19.45, -6.25) -> (23.55, -6.25) centre (21.5, -6.25) ccw construction
  line L4 (23.55, 6.25) -> (23.55, -6.25) construction
  arc A3 (23.55, 6.25) -> (19.45, 6.25) centre (21.5, 6.25) ccw construction
  line L5 (21.5, -6.25) -> (21.5, 6.25) construction
  constraints: 4 end point, 2 vertical
body "Solid3"
